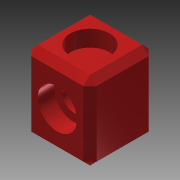
# Autodesk Inventor part: piece roulement
Saved by Autodesk Inventor 2015 (Build 190159000, 159)
## iProperties
Created: 2014-12-21
Part Number: piece roulement
Material: Générique
Document SubType Name: Modeling
Designer: emield
Density: 1 g/cm^3
Appearance: Rouge clair
Author: emield
Autodesk Inventor part; units mm, degrees
ref_plane "YZ Plane" through (0, 0, 0) normal (1, 0, 0) x (0, 1, 0)
ref_plane "XZ Plane" through (0, 0, 0) normal (0, 1, 0) x (-1, 0, 0)
ref_plane "XY Plane" through (0, 0, 0) normal (0, 0, 1) x (1, 0, 0)
sketch "Esquisse1" plane through (0, 0, 0) normal (0, 1, 0) x (-1, 0, 0)
  line L0 (5, 6) -> (-5, 6)
  line L1 (-5, 6) -> (-5, -6)
  line L2 (-5, -6) -> (5, -6)
  line L3 (5, -6) -> (5, 6)
  point P0 (0, 0)
  dimension "d0" = 10
  dimension "d1" = 5
  dimension "d2" = 6
  dimension "d3" = 6
  constraints: 8 end point, 2 parallel, 1 horizontal, 1 perpendicular
  measures "d0" distance of L1.end L2.end
  measures "d1" distance from line of L1 point (0, 0)
  measures "d2" distance from line of L0 point (0, 0)
  measures "d3" distance from line of point (0, 0) L2
extrude "Extrusion1" add sketch "Esquisse1" along normal blind 10
sketch "Esquisse2" plane through (-5, 0, 6) normal (0, 0, 1) x (1, 0, 0)
  circle A0 centre (5, 5) radius 3
  line L0 (0, 0) -> (0, 10) projected
  point P0 (5, 0)
  dimension "d6" = 6
  dimension "d7" = 5
  dimension "d8" = 5
  constraints: 1 centre point
  measures "d6" diameter of A0
  measures "d7" distance of point (5, 0) A0.centre
  measures "d8" distance from line of A0.centre L0
extrude "Extrusion2" cut sketch "Esquisse2" against normal blind 2.5
sketch "Esquisse3" plane through (5, 0, -6) normal (0, 0, -1) x (-1, 0, 0)
  circle A0 centre (5, 5) radius 3 projected
  point P0 (5, 0)
extrude "Extrusion3" cut sketch "Esquisse3" against normal blind 2.5
sketch "Esquisse4" plane through (0, 0, 0) normal (0, -1, 0) x (1, 0, 0)
  circle A0 centre (0, 0) radius 3
  dimension "d13" = 6
  constraints: 1 centre point, 1 coincident
  measures "d13" diameter of A0
extrude "Extrusion4" cut sketch "Esquisse4" against normal blind 2.5
sketch "Esquisse5" plane through (0, 10, 0) normal (0, 1, 0) x (1, 0, 0)
  circle A0 centre (0, 0) radius 3 projected
  circle A1 centre (0, 0) radius 3 projected
extrude "Extrusion5" cut sketch "Esquisse5" against normal blind 2.5
sketch "Esquisse6" plane through (0, 7.5, 0) normal (0, 1, 0) x (1, 0, 0)
  circle A0 centre (0, 0) radius 1.75
  dimension "d18" = 3.5
  constraints: 1 centre point, 1 coincident
  measures "d18" diameter of A0
extrude "Extrusion6" cut sketch "Esquisse6" against normal up to surface (5 mm away)
chamfer "Chanfrein1" distance 1 angle 45 12 edges at (5, 10, 0) (0, 10, 6) (5, 5, 6) (-5, 5, 6) (0, 0, 6) (5, 0, 0) (5, 5, -6) (0, 0, -6) (-5, 0, 0) (-5, 10, 0) (0, 10, -6) (-5, 5, -6)
